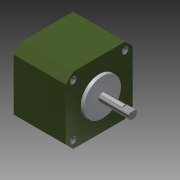
# Autodesk Inventor part: Stepper_Motor
Saved by Autodesk Inventor 2014 (Build 180170000, 170)
## iProperties
Created: 2014-11-07
Part Number: Stepper_Motor
Material: Generic
Document SubType Name: Modeling
Designer: nfitch
Density: 1 g/cm^3
Appearance: Default
Author: nfitch
Autodesk Inventor part; units mm, degrees
ref_plane "YZ Plane" through (0, 0, 0) normal (1, 0, 0) x (0, 1, 0)
ref_plane "XZ Plane" through (0, 0, 0) normal (0, 1, 0) x (-1, 0, 0)
ref_plane "XY Plane" through (0, 0, 0) normal (0, 0, 1) x (1, 0, 0)
sketch "Sketch1" plane through (0, 0, 0) normal (1, 0, 0) x (0, 1, 0)
  line L0 (-20, 20) -> (20, 20)
  line L1 (20, 20) -> (20, -20)
  line L2 (20, -20) -> (-20, -20)
  line L3 (-20, -20) -> (-20, 20)
  line L4 (-20, 20) -> (20, -20) construction
  line L5 (20, 20) -> (-20, -20) construction
  point P0 (0, 0)
  point P1 (0, 0)
  dimension "d0" = 40
  dimension "d1" = 40
  constraints: 12 end point, 2 midpoint, 2 parallel, 1 horizontal, 1 perpendicular
  measures "d0" distance of L1.end L2.end
  measures "d1" distance of L0.end L1.end
extrude "Extrusion1" add sketch "Sketch1" along normal blind 33
sketch "Sketch2" plane through (33, 0, 0) normal (1, 0, 0) x (0, 0, -1)
  line L0 (-20, 20) -> (-20, -20) projected
  line L1 (-20, -20) -> (20, -20) projected
  line L2 (20, -20) -> (20, 20) projected
  line L3 (20, 20) -> (-20, 20) projected
  circle A0 centre (0, 0) radius 11
  dimension "d4" = 22
  constraints: 1 centre point
  measures "d4" diameter of A0
extrude "Extrusion2" cut sketch "Sketch2" against normal blind 2
sketch "Sketch3" plane through (33, 0, 0) normal (1, 0, 0) x (0, 0, -1)
  circle A0 centre (0, 0) radius 2.5
  dimension "d7" = 5
  constraints: 1 centre point
  measures "d7" diameter of A0
extrude "Extrusion3" add sketch "Sketch3" along normal blind 18
sketch "Sketch4" plane through (31, 0, 0) normal (1, 0, 0) x (0, 0, -1)
  line L0 (20, 20) -> (20, -20) projected
  line L1 (-20, 20) -> (20, 20) projected
  point P0 (15.5, 15.5)
  point P1 (-15.5, 15.5)
  point P2 (15.5, -15.5)
  point P3 (-15.5, -15.5)
  dimension "d12" = 31
  dimension "d15" = 31
  constraints: 1 horizontal, 1 vertical, 3 other
  measures "d12" distance of point (15.5, 15.5) point (-15.5, 15.5)
  measures "d15" distance of point (15.5, 15.5) point (15.5, -15.5)
hole "Hole1" at (31, 15.5, -15.5) at (31, 15.5, 15.5) at (31, -15.5, -15.5) at (31, -15.5, 15.5) direction (-1, 0, 0) diameter 2.459 end through all countersink diameter 4 countersink angle 90 thread size "M3x0.5" class "6H" standard "ANSI Metric M Profile"
chamfer "Chamfer1" distance 4.5 angle 45 4 edges at (15.5, 20, -20) (15.5, -20, -20) (15.5, 20, 20) (15.5, -20, 20)
sketch "Sketch7" plane through (51, 0, 0) normal (1, 0, 0) x (0, 0, -1)
  line L0 (-2.5, 1.7499) -> (2.5, 1.7499)
  line L1 (2.5, 1.7499) -> (2.5, 3.2499)
  line L2 (2.5, 3.2499) -> (-2.5, 3.2499)
  line L3 (-2.5, 3.2499) -> (-2.5, 1.7499)
  line L4 (-2.5, 1.7499) -> (2.5, 3.2499) construction
  line L5 (2.5, 1.7499) -> (-2.5, 3.2499) construction
  point P0 (0, 2.4999)
  dimension "d29" = 5
  dimension "d30" = 1.5
  constraints: 12 end point, 2 midpoint, 2 parallel, 1 horizontal, 1 perpendicular
  measures "d29" distance of L2.end L1.end
  measures "d30" distance of L1.end L0.end
extrude "Extrusion4" cut sketch "Sketch7" against normal blind 5
body "Solid1"
